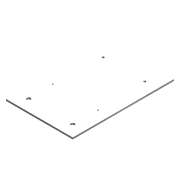
# Autodesk Inventor part: SupportsheetStandard2
Saved by Autodesk Inventor 2017 (Build 210142000, 142)
## iProperties
Created: 2016-11-07
Part Number: SupportsheetStandard2
Material: Aluminum 6061
Document SubType Name: Modeling
Designer: Jonis
Density: 2.7 g/cm^3
Appearance: Aluminum - Flat
Author: Jonis
Autodesk Inventor part; units mm, degrees
ref_plane "YZ Plane" through (0, 0, 0) normal (1, 0, 0) x (0, 1, 0)
ref_plane "XZ Plane" through (0, 0, 0) normal (0, 1, 0) x (-1, 0, 0)
ref_plane "XY Plane" through (0, 0, 0) normal (0, 0, 1) x (1, 0, 0)
sketch "Sketch1" plane through (0, 0, 0) normal (0, 1, 0) x (-1, 0, 0)
  line L0 (0, 0) -> (118, 0)
  line L1 (118, 0) -> (118, -179)
  line L2 (118, -179) -> (0, -179)
  line L3 (0, -179) -> (0, 0)
  dimension "d0" = 118
  dimension "d1" = 179
  constraints: 8 end point, 2 parallel, 1 horizontal, 1 perpendicular
  measures "d0" distance of L1.end L2.end
  measures "d1" distance of L0.end L1.end
extrude "Extrusion1" add sketch "Sketch1" along normal blind 3
sketch "Sketch2" plane through (0, 3, 0) normal (0, 1, 0) x (1, 0, 0)
  line L0 (-118, 0) -> (0, 0) projected
  line L1 (0, 0) -> (0, 179) projected
  line L2 (-118, 179) -> (-118, 0) projected
  point P0 (-20, 20)
  point P1 (-98, 20)
  dimension "d4" = 20
  dimension "d5" = 20
  dimension "d6" = 20
  dimension "d7" = 20
  measures "d4" distance from line of point (-20, 20) L0
  measures "d5" distance from line of point (-20, 20) L1
  measures "d6" distance from line of L0 point (-98, 20)
  measures "d7" distance from line of point (-98, 20) L2
hole "Hole1" at (-20, 3, -20) at (-98, 3, -20) direction (0, -1, 0) diameter 7 end through all
sketch "Sketch9" plane through (0, 3, 0) normal (0, 1, 0) x (1, 0, 0)
  circle A0 centre (-14.5, 117) radius 1.6
  circle A1 centre (-14.5, 41) radius 1.6
  circle A2 centre (-20, 20) radius 3.5 projected
  circle A3 centre (-98, 20) radius 3.5 projected
  line L0 (-118, 0) -> (0, 0) projected
  line L1 (0, 0) -> (0, 179) projected
  line L2 (0, 179) -> (-118, 179) projected
  line L3 (-118, 179) -> (-118, 0) projected
  circle A4 centre (-103.5, 117) radius 1.6
  circle A5 centre (-103.5, 41) radius 1.6
  circle A6 centre (-22.17, 145.87) radius 1.75
  circle A7 centre (-95.83, 145.87) radius 1.75
  dimension "d68" = 33.13
  dimension "d69" = 33.13
  dimension "d70" = 62
  dimension "d71" = 138
  dimension "d72" = 14.5
  dimension "d73" = 14.5
  dimension "d74" = 22.17
  dimension "d75" = 95.83
  constraints: 6 centre point, 12 other
  measures "d68" distance from line of A7.centre L2
  measures "d69" distance from line of A6.centre L2
  measures "d70" distance from line of A0.centre L2
  measures "d71" distance from line of A1.centre L2
  measures "d72" distance from line of A4.centre L3
  measures "d73" distance from line of A5.centre L3
  measures "d74" distance from line of A7.centre L3
  measures "d75" distance from line of A6.centre L3
body "Solid1"
